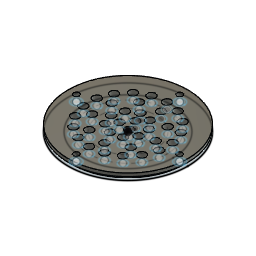
57mm speaker grill v1.0 (Autodesk Fusion 360 design; units mm, degrees)
Autodesk Fusion 360 part; units mm, degrees
sketch "Sketch1" plane through (0, 0, 0) normal (0, 1, 0) x (1, 0, 0)
  circle A0 centre (0, 0) radius 37
  circle A1 centre (0.0545, 32.013) radius 1.75
  circle A2 centre (-32.013, 0.0545) radius 1.75
  circle A3 centre (-0.0545, -32.013) radius 1.75
  circle A4 centre (32.013, -0.0545) radius 1.75
  circle A5 centre (0, 0) radius 28
  circle A6 centre (0, 0) radius 24 construction
  circle A7 centre (0.1333, 23.9996) radius 2.5 construction
  circle A8 centre (0, 0) radius 17.5 construction
  circle A9 centre (0, 0) radius 10 construction
  circle A10 centre (0, 0) radius 4 construction
  circle A11 centre (0.1333, 23.9996) radius 2.5
  circle A12 centre (-8.0831, 22.5979) radius 2.5
  circle A13 centre (-15.3245, 18.4705) radius 2.5
  circle A14 centre (-20.7176, 12.1153) radius 2.5
  circle A15 centre (-23.6119, 4.2988) radius 2.5
  circle A16 centre (-23.6582, -4.0362) radius 2.5
  circle A17 centre (-20.851, -11.8843) radius 2.5
  circle A18 centre (-15.5288, -18.2991) radius 2.5
  circle A19 centre (-8.3337, -22.5067) radius 2.5
  circle A20 centre (-0.1333, -23.9996) radius 2.5
  circle A21 centre (8.0831, -22.5979) radius 2.5
  circle A22 centre (15.3245, -18.4705) radius 2.5
  circle A23 centre (20.7176, -12.1153) radius 2.5
  circle A24 centre (23.6119, -4.2988) radius 2.5
  circle A25 centre (23.6582, 4.0362) radius 2.5
  circle A26 centre (20.851, 11.8843) radius 2.5
  circle A27 centre (15.5288, 18.2991) radius 2.5
  circle A28 centre (8.3337, 22.5067) radius 2.5
  circle A29 centre (3.3532, 17.1757) radius 2.5
  circle A30 centre (-8.4717, 15.3128) radius 2.5
  circle A31 centre (-16.3325, 6.2848) radius 2.5
  circle A32 centre (-16.5512, -5.6839) radius 2.5
  circle A33 centre (-9.0254, -14.9931) radius 2.5
  circle A34 centre (2.7235, -17.2868) radius 2.5
  circle A35 centre (13.198, -11.4918) radius 2.5
  circle A36 centre (17.4971, -0.3197) radius 2.5
  circle A37 centre (13.609, 11.002) radius 2.5
  circle A38 centre (-2.1579, 9.7644) radius 2.5
  circle A39 centre (-7.9295, 6.0929) radius 2.5
  circle A40 centre (-9.9908, -0.4296) radius 2.5
  circle A41 centre (-7.3772, -6.751) radius 2.5
  circle A42 centre (-1.3118, -9.9136) radius 2.5
  circle A43 centre (5.3674, -8.4375) radius 2.5
  circle A44 centre (9.5352, -3.0134) radius 2.5
  circle A45 centre (9.2413, 3.8207) radius 2.5
  circle A46 centre (4.6234, 8.867) radius 2.5
  circle A47 centre (0.4427, 3.9754) radius 2.5
  circle A48 centre (-3.6642, -1.6043) radius 2.5
  circle A49 centre (3.2214, -2.3711) radius 2.5
  circle A50 centre (0.0545, 32.013) radius 3
  circle A51 centre (32.013, -0.0545) radius 3
  circle A52 centre (-0.0545, -32.013) radius 3
  circle A53 centre (-32.013, 0.0545) radius 3
  dimension "d2" = 74
  dimension "d3" = 3.5
  dimension "d5" = 360
  dimension "d8" = 56
  dimension "d11" = 48
  dimension "d12" = 5
  dimension "d13" = 35
  dimension "d14" = 20
  dimension "d15" = 8
  dimension "d16" = 5
  dimension "d18" = 360
  dimension "d19" = 5
  dimension "d21" = 360
  dimension "d22" = 5
  dimension "d24" = 360
  dimension "d25" = 5
  dimension "d27" = 360
  dimension "d30" = 6
  dimension "d31" = 6
  dimension "d32" = 6
  dimension "d33" = 6
  constraint coincident A0.centre A5.centre
  constraint concentric A5 A6
  constraint coincident A6 A7.centre
  constraint concentric A0 A8
  constraint concentric A8 A9
  constraint concentric A9 A10
  constraint concentric A7 A11
  constraint coincident A8 A29.centre
  constraint coincident A9 A38.centre
  constraint coincident A10 A47.centre
  constraint concentric A1 A50
  constraint concentric A4 A51
  constraint concentric A3 A52
  constraint concentric A2 A53
  measures "d2" diameter of A0
  measures "d3" diameter of A1
  measures "d8" diameter of A5
  measures "d11" diameter of A6
  measures "d12" diameter of A7
  measures "d13" diameter of A8
  measures "d14" diameter of A9
  measures "d15" diameter of A10
  measures "d16" diameter of A11
  measures "d19" diameter of A29
  measures "d22" diameter of A38
  measures "d25" diameter of A47
  measures "d30" diameter of A50
  measures "d31" diameter of A51
  measures "d32" diameter of A52
  measures "d33" diameter of A53
extrude "Extrude1" add sketch "Sketch1" along normal blind 4 contours A0 | A5 | A11 | A12 | A13 | A14 | A15 | A16 | A17 | A18 | A19 | A20 | A21 | A22 | A23 | A24 | A25 | A26 | A27 | A28 | A29 | A30 | A31 | A32 | A33 | A34 | A35 | A36 | A37 | A38 | A39 | A40 | A41 | A42 | A43 | A44 | A45 | A46 | A47 | A48 | A49 | A50 | A51 | A52 | A53
extrude "Extrude3" cut sketch "Sketch1" along normal up to surface (4 mm away) contours A11 | A12 | A13 | A14 | A15 | A16 | A17 | A18 | A19 | A20 | A21 | A22 | A23 | A24 | A25 | A26 | A27 | A28 | A29 | A30 | A31 | A32 | A33 | A34 | A35 | A36 | A37 | A38 | A39 | A40 | A41 | A42 | A43 | A44 | A45 | A46 | A47 | A48 | A49
extrude "Extrude4" cut sketch "Sketch1" along normal blind 1.5 contours A50 | A51 | A52 | A53
chamfer "Chamfer1" distance 2 angle 45 1 edges at (-34.4961, 0, 13.3798)
